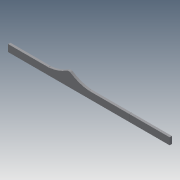
# Autodesk Inventor part: packa_sablona_jekl
Saved by Autodesk Inventor 2013 (Build 170138000, 138)
## iProperties
Created: 2013-06-15
Part Number: packa_sablona_jekl
Material: Generic
Document SubType Name: Modeling
Designer: idle-rug
Density: 1 g/cm^3
Author: idle-rug
Autodesk Inventor part; units mm, degrees
ref_plane "YZ Plane" through (0, 0, 0) normal (1, 0, 0) x (0, 1, 0)
ref_plane "XZ Plane" through (0, 0, 0) normal (0, 1, 0) x (-1, 0, 0)
ref_plane "XY Plane" through (0, 0, 0) normal (0, 0, 1) x (1, 0, 0)
sketch "Sketch1" plane through (0, 0, 0) normal (0, 1, 0) x (-1, 0, 0)
  line L0 (-70, 3) -> (-70, -3)
  line L1 (-70, -3) -> (70, -3)
  line L2 (70, -3) -> (70, 3)
  line L3 (-70, 3) -> (-35, 3)
  line L4 (-35, 3) -> (-35, -3)
  line L5 (0, 3) -> (0, -3)
  line L6 (0, 3) -> (35, 3)
  line L7 (35, 3) -> (35, -3)
  line L8 (-34.9, 3) -> (-34.9, -3)
  line L9 (-34.9, -3) -> (-35, -3)
  line L10 (-0.1, 3) -> (-0.1, -3)
  line L11 (-0.1, -3) -> (0, -3)
  line L12 (35.1, 3) -> (35.1, -3)
  line L13 (35.1, -3) -> (35, -3)
  line L14 (0, 0) -> (35, 0)
  arc A0 (19.1361, 8.5146) -> (35, 3) centre (38.2245, 37.8512) ccw
  arc A1 (0, 3) -> (15.8639, 8.5146) centre (-3.2245, 37.8512) ccw
  circle A2 centre (17.5, 6) radius 0.05
  circle A3 centre (17.5, 0) radius 0.05
  line L15 (70, 3) -> (35.1, 3)
  arc A4 (19.1361, 8.5146) -> (15.8639, 8.5146) centre (17.5, 6) ccw
  line L16 (70, 3) -> (35.1, 3)
  line L17 (35.1, 2.988) -> (35.1, -3)
  line L18 (35.1, -3) -> (70, -3)
  line L19 (70, -3) -> (70, 3)
  line L20 (-0.1, 3) -> (-34.9, 3)
  line L21 (35, 3) -> (0, 3)
  dimension "d0" = 140
  dimension "d1" = 6
  dimension "d2" = 35
  dimension "d3" = 35
  dimension "d4" = 35
  dimension "d5" = 0.1
  dimension "d6" = 6
  dimension "d7" = 0.1
  dimension "d8" = 6
  dimension "d9" = 0.1
  dimension "d10" = 6
  constraints: 44 end point, 6 point on circle, 5 centre point, 5 point on line, 4 collinear, 4 perpendicular, 2 midpoint, 1 parallel, 1 tangent
  measures "d0" distance of L1.end L0.end
  measures "d1" distance of L0.start L0.end
  measures "d2" distance of L0.start L3.end
  measures "d3" distance of L3.end L5.start
  measures "d4" distance of L5.start L6.end
  measures "d5" distance of L3.end L8.start
  measures "d6" distance of L8.start L8.end
  measures "d7" distance of L5.start L10.start
  measures "d8" distance of L10.start L10.end
  measures "d9" distance of L6.end L12.start
  measures "d10" distance of L12.start L12.end
extrude "Extrusion1" add sketch "Sketch1" along normal blind 2 contours L3 L4 L1 L0 | L12 L15 L2 L1 | L5 L14 A3 L7 L1 | L8 L20 L10 L1 | L5 L6 L7 L14 A3 | A1 A4 A0 L6
body "Solid1"
